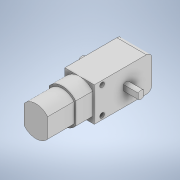
# Autodesk Inventor part: мотор лол
Saved by Autodesk Inventor 2021.2 (Build 252289000, 289)
## iProperties
Created: 2022-07-09
Part Number: мотор лол
Material: Типовые
Document SubType Name: Modeling
Designer: ROOT
Density: 1 g/cm^3
Appearance: По умолчанию
Author: ROOT
Autodesk Inventor part; units mm, degrees
ref_plane "YZ Plane" through (0, 0, 0) normal (1, 0, 0) x (0, 1, 0)
ref_plane "XZ Plane" through (0, 0, 0) normal (0, 1, 0) x (-1, 0, 0)
ref_plane "XY Plane" through (0, 0, 0) normal (0, 0, 1) x (1, 0, 0)
sketch "Эскиз1" plane through (0, 0, 0) normal (0, 0, 1) x (1, 0, 0)
  line L0 (9.5, -11) -> (-9.5, -11)
  line L1 (-9.5, -11) -> (-9.5, 11)
  line L2 (-9.5, 11) -> (9.5, 11)
  line L3 (9.5, 11) -> (9.5, -11)
  line L4 (9.5, -11) -> (-9.5, 11) construction
  line L5 (-9.5, -11) -> (9.5, 11) construction
  point P0 (0, 0)
  dimension "d0" = 19
  dimension "d1" = 22
  constraints: 12 end point, 2 midpoint, 2 parallel, 1 horizontal, 1 perpendicular
  measures "d0" distance of L1.end L2.end
  measures "d1" distance of L0.end L1.end
extrude "Выдавливание1" add sketch "Эскиз1" along normal blind 37
sketch "Эскиз2" plane through (0, 0, 37) normal (0, 0, 1) x (1, 0, 0)
  circle A0 centre (0, 0) radius 11
  line L0 (8.5, -20.0649) -> (-8.5, -20.0649)
  line L1 (-8.5, -20.0649) -> (-8.5, 20.0649)
  line L2 (-8.5, 20.0649) -> (8.5, 20.0649)
  line L3 (8.5, 20.0649) -> (8.5, -20.0649)
  line L4 (8.5, -20.0649) -> (-8.5, 20.0649) construction
  line L5 (-8.5, -20.0649) -> (8.5, 20.0649) construction
  point P0 (8.5, -6.9821)
  point P1 (8.5, 6.9821)
  point P2 (-8.5, 6.9821)
  point P3 (-8.5, -6.9821)
  dimension "d4" = 22
  dimension "d5" = 17
  constraints: 12 end point, 2 midpoint, 2 parallel, 1 centre point, 1 coincident, 1 horizontal, 1 perpendicular
  measures "d4" diameter of A0
  measures "d5" distance of L1.end L2.end
extrude "Выдавливание2" add sketch "Эскиз2" along normal blind 11 contours L3 A0 L1
sketch "Эскиз3" plane through (9.5, -11, 0) normal (1, 0, 0) x (0, 0, -1)
  circle A0 centre (-32, 19.5) radius 1.5
  line L0 (-37, 0) -> (-37, 22) projected
  line L1 (0, 22) -> (-37, 22) projected
  line L2 (-37, 4.0179) -> (-37, 17.9821) projected
  line L3 (-37, 11) -> (0, 11)
  line L4 (0, 0) -> (0, 22) projected
  circle A1 centre (-32, 2.5) radius 1.5
  dimension "d8" = 3
  dimension "d9" = 5
  dimension "d10" = 2.5
  constraints: 2 centre point, 2 end point, 1 midpoint, 1 perpendicular, 1 symmetric about line, 1 other
  measures "d8" diameter of A0
  measures "d9" distance from line of L0 A0.centre
  measures "d10" distance from line of L1 A0.centre
extrude "Выдавливание3" cut sketch "Эскиз3" against normal through all contours A0 | A1
sketch "Эскиз4" plane through (9.5, -11, 0) normal (1, 0, 0) x (0, 0, -1)
  circle A0 centre (-16.5, 11) radius 2.5
  line L0 (0, 0) -> (0, 22) projected
  line L1 (0, 0) -> (-37, 0) projected
  line L2 (-14.75, 6.8216) -> (-18.25, 6.8216)
  line L3 (-18.25, 6.8216) -> (-18.25, 15.1784)
  line L4 (-18.25, 15.1784) -> (-14.75, 15.1784)
  line L5 (-14.75, 15.1784) -> (-14.75, 6.8216)
  line L6 (-14.75, 6.8216) -> (-18.25, 15.1784) construction
  line L7 (-18.25, 6.8216) -> (-14.75, 15.1784) construction
  point P0 (0, 11)
  point P1 (-14.75, 9.2146)
  point P2 (-14.75, 12.7854)
  point P3 (-18.25, 12.7854)
  point P4 (-18.25, 9.2146)
  dimension "d13" = 5
  dimension "d14" = 16.5
  dimension "d15" = 11
  dimension "d16" = 3.5
  constraints: 12 end point, 2 midpoint, 2 parallel, 1 centre point, 1 horizontal, 1 perpendicular
  measures "d13" diameter of A0
  measures "d14" distance from line of L0 A0.centre
  measures "d15" distance from line of L1 A0.centre
  measures "d16" distance of L3.end L4.end
extrude "Выдавливание4" add sketch "Эскиз4" along normal blind 9.5 and the other way blind 28.5 contours L5 A0 L3
sketch "Эскиз5" plane through (0, 0, 48) normal (0, 0, 1) x (1, 0, 0)
  circle A0 centre (0, 0) radius 9.75
  line L0 (7.5, 17.2473) -> (-7.5, 17.2473)
  line L1 (-7.5, 17.2473) -> (-7.5, -17.2473)
  line L2 (-7.5, -17.2473) -> (7.5, -17.2473)
  line L3 (7.5, -17.2473) -> (7.5, 17.2473)
  line L4 (7.5, 17.2473) -> (-7.5, -17.2473) construction
  line L5 (-7.5, 17.2473) -> (7.5, -17.2473) construction
  point P0 (7.5, -6.23)
  point P1 (7.5, 6.23)
  point P2 (-7.5, 6.23)
  point P3 (-7.5, -6.23)
  dimension "d21" = 19.5
  dimension "d22" = 15
  constraints: 12 end point, 2 midpoint, 2 parallel, 1 centre point, 1 coincident, 1 horizontal, 1 perpendicular
  measures "d21" diameter of A0
  measures "d22" distance of L0.start L0.end
extrude "Выдавливание5" add sketch "Эскиз5" along normal blind 17 contours L3 A0 L1
fillet "Сопряжение1" radius 3.5 2 edges at (0, -11, 0) (0, 11, 0)
sketch "Эскиз6" plane through (0, 0, 0) normal (0, 0, -1) x (-1, 0, 0)
  line L0 (-1.25, 2.5) -> (1.25, 2.5)
  line L1 (1.25, 2.5) -> (1.25, -2.5)
  line L2 (1.25, -2.5) -> (-1.25, -2.5)
  line L3 (-1.25, -2.5) -> (-1.25, 2.5)
  line L4 (-1.25, 2.5) -> (1.25, -2.5) construction
  line L5 (1.25, 2.5) -> (-1.25, -2.5) construction
  point P0 (0, 0)
  dimension "d26" = 2.5
  dimension "d27" = 5
  constraints: 12 end point, 2 midpoint, 2 parallel, 1 horizontal, 1 perpendicular
  measures "d26" distance of L1.end L2.end
  measures "d27" distance of L2.end L0.start
extrude "Выдавливание6" add sketch "Эскиз6" along normal blind 4.5
sketch "Эскиз7" plane through (-1.25, -2.5, 0) normal (-1, 0, 0) x (0, 0, 1)
  line L0 (0, 0) -> (-4.5, 0) projected
  line L1 (0, 5) -> (-4.5, 5) projected
  line L2 (-4.5, 0) -> (-4.5, 5) projected
  line L3 (-4.5, 2.5) -> (0, 2.5)
  circle A0 centre (-2.25, 2.5) radius 1.5
  dimension "d31" = 3
  constraints: 2 end point, 2 midpoint, 1 centre point, 1 horizontal
  measures "d31" diameter of A0
extrude "Выдавливание7" cut sketch "Эскиз7" against normal through all
